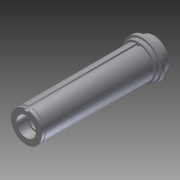
# Autodesk Inventor part: turn shaft 2
Saved by Autodesk Inventor 2012 (Build 160160000, 160)
## iProperties
Created: 2012-07-19
Part Number: turn shaft 2
Material: Default
Document SubType Name: Modeling
Designer: Team-2471
Density: 1 g/cm^3
Author: Team-2471
Autodesk Inventor part; units mm, degrees
sketch "Sketch1" plane through (0, 0, 0) normal (0, 0, 1) x (1, 0, 0)
  circle A0 centre (0, 0) radius 12.7
  circle A1 centre (0, 0) radius 6.35
  line L0 (-1.5875, 14.2875) -> (1.5875, 14.2875)
  line L1 (1.5875, 14.2875) -> (1.5875, 11.1125)
  line L2 (1.5875, 11.1125) -> (-1.5875, 11.1125)
  line L3 (-1.5875, 11.1125) -> (-1.5875, 14.2875)
  dimension "d0" = 25.4
  dimension "d4" = 12.7
  dimension "d50" = 3.175
  dimension "d51" = 3.175
  dimension "d52" = 1.5875
  dimension "d53" = 14.2875
  constraints: 8 end point, 2 centre point, 2 parallel, 1 coincident, 1 concentric, 1 horizontal, 1 perpendicular
  measures "d0" diameter of A0
  measures "d4" diameter of A1
  measures "d50" distance of L0.start L0.end
  measures "d51" distance of L0.end L1.end
  measures "d52" distance from line of L1 point (0, 0)
  measures "d53" distance from line of point (0, 0) L0
extrude "Extrusion4" add sketch "Sketch1" along normal blind 104.775 contours A0 L3 L2 L1 | L1 L2 L3 A0
ref_plane "Work Plane5" through (0, 0, 101.6) normal (0, 0, 1) x (1, 0, 0)
sketch "Sketch6" plane through (0, 0, 101.6) normal (0, 0, 1) x (1, 0, 0)
  circle A0 centre (0, 0) radius 12.192
  circle A1 centre (0, 0) radius 12.7 projected
  dimension "d24" = 24.384
  constraints: 1 centre point, 1 coincident
  measures "d24" diameter of A0
extrude "Extrusion8" cut sketch "Sketch6" along normal blind 1.143
ref_plane "Work Plane6" through (0, 0, 15.113) normal (0, 0, -1) x (-1, 0, 0)
ref_plane "Work Plane9" through (0, 0, 43.3324) normal (0, 0, -1) x (-1, 0, 0)
ref_plane "Work Plane10" through (0, 0, 29.464) normal (0, 0, -1) x (-1, 0, 0)
extrude "Extrusion16" cut sketch "Sketch1" along normal through all contours L1 L2 L3 A0 | A0 L3 L0 L1 picked at (0.1768, 11.638)
sketch "Sketch14" plane through (0, 0, 104.775) normal (0, 0, 1) x (1, 0, 0)
  circle A0 centre (0, 0) radius 6.35 projected
  circle A1 centre (0, 0) radius 7.9375
  dimension "d56" = 15.875
  constraints: 1 centre point, 1 coincident
  measures "d56" diameter of A1
extrude "Extrusion17" cut sketch "Sketch14" against normal blind 7.9375
sketch "Sketch15" plane through (0, 0, 0) normal (0, 0, -1) x (-1, 0, 0)
  circle A0 centre (0, 0) radius 6.35 projected
  circle A1 centre (0, 0) radius 7.9375
  dimension "d59" = 15.875
  constraints: 1 centre point, 1 coincident
  measures "d59" diameter of A1
extrude "Extrusion18" cut sketch "Sketch15" against normal blind 7.9375
ref_plane "Work Plane13" through (0, 0, 6.35) normal (0, 0, -1) x (-1, 0, 0)
sketch "Sketch16" plane through (0, 0, 6.35) normal (0, 0, -1) x (-1, 0, 0)
  arc A0 (-1.5875, 12.6004) -> (1.5875, 12.6004) centre (0, 0) ccw projected
  line L0 (-1.5875, 12.6004) -> (-1.5875, 11.1125) projected
  line L1 (-1.5875, 11.1125) -> (1.5875, 11.1125) projected
  line L2 (1.5875, 11.1125) -> (1.5875, 12.6004) projected
  circle A1 centre (0, 0) radius 15.875
  circle A2 centre (0, 0) radius 14.2875
  dimension "d63" = 31.75
  dimension "d68" = 28.575
  constraints: 2 centre point, 2 coincident
  measures "d63" diameter of A1
  measures "d68" diameter of A2
extrude "Extrusion19" add sketch "Sketch16" against normal blind 3.175 contours A1 | A2
sketch "Sketch17" plane through (0, 0, 0) normal (0, 0, -1) x (-1, 0, 0)
  line L0 (-1.5875, 11.1125) -> (-1.5875, 12.6004) projected
  arc A0 (-1.5875, 12.6004) -> (1.5875, 12.6004) centre (0, 0) ccw projected
  line L1 (1.5875, 12.6004) -> (1.5875, 11.1125) projected
  line L2 (1.5875, 11.1125) -> (-1.5875, 11.1125) projected
  arc A1 (1.5875, 12.6004) -> (-1.5875, 12.6004) centre (0, 0) ccw
  constraints: 2 point on circle, 1 centre point, 1 coincident
extrude "Extrusion20" add sketch "Sketch17" against normal blind 6.35 contours L0 A1 L1 L2
extrude "Extrusion21" add sketch "Sketch16" against normal blind 6.35 contours A2
equation "\"d51\" = d50"
equation "\"d52\" = 0.5 * d50"
equation "\"d53\" = 0.5 * d0 + 0.5 * d50"
body "Solid2"
